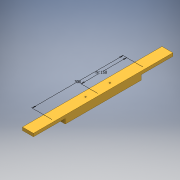
# Autodesk Inventor part: piXYstageStiltAttach
Saved by Autodesk Inventor 2016 (Build 200138000, 138)
## iProperties
Created: 2016-03-15
Part Number: piXYstageStiltAttach
Material: Generic
Document SubType Name: Modeling
Designer: sims01
Density: 1 g/cm^3
Appearance: Default
Author: sims01
Autodesk Inventor part; units mm, degrees
ref_plane "YZ Plane" through (0, 0, 0) normal (1, 0, 0) x (0, 1, 0)
ref_plane "XZ Plane" through (0, 0, 0) normal (0, 1, 0) x (-1, 0, 0)
ref_plane "XY Plane" through (0, 0, 0) normal (0, 0, 1) x (1, 0, 0)
sketch "Sketch1" plane through (0, 0, 0) normal (0, 0, 1) x (1, 0, 0)
  line L0 (-8, 55.5375) -> (8, 55.5375)
  line L1 (8, 55.5375) -> (8, -55.5375)
  line L2 (8, -55.5375) -> (-8, -55.5375)
  line L3 (-8, -55.5375) -> (-8, 55.5375)
  line L4 (-18, 229.9628) -> (18, 229.9628)
  line L5 (18, 229.9628) -> (18, -229.9628)
  line L6 (18, -229.9628) -> (-18, -229.9628)
  line L7 (-18, -229.9628) -> (-18, 229.9628)
  point P0 (0, 0)
  dimension "d0" = 16
  dimension "d1" = 111.075
  dimension "d2" = 55.5375
  dimension "d3" = 8
  dimension "d6" = 10
  dimension "d7" = 174.4253
  dimension "d8" = 10
  dimension "d9" = 174.4253
  constraints: 16 end point, 4 parallel, 2 horizontal, 2 perpendicular
  measures "d0" distance of L0.start L0.end
  measures "d1" distance of L0.end L1.end
  measures "d2" distance from line of point (0, 0) L0
  measures "d3" distance from line of point (0, 0) L1
  measures "d6" distance between parallel lines of L7 L3
  measures "d7" distance between parallel lines of L0 L4
  measures "d8" distance between parallel lines of L5 L1
  measures "d9" distance between parallel lines of L6 L2
sketch "Sketch2" plane through (0, 0, 0) normal (0, 0, 1) x (1, 0, 0)
  point P0 (0, 0)
  point P1 (0, 40)
  point P2 (0, -40)
  dimension "d4" = 80
  dimension "d5" = 40
  constraints: 2 vertical alignment
  measures "d4" distance of point (0, -40) point (0, 40)
  measures "d5" distance of point (0, 0) point (0, 40)
sketch "Sketch3" plane through (0, 0, 0) normal (0, 0, 1) x (1, 0, 0)
  point P0 (0, 0)
  point P1 (0, -150)
  point P2 (0, 150)
  dimension "d10" = 300
  dimension "d11" = 150
  constraints: 2 vertical alignment
  measures "d10" distance of point (0, 150) point (0, -150)
  measures "d11" distance of point (0, 0) point (0, 150)
extrude "baseExtrusion" add sketch "Sketch1" along normal blind 10 contours L0 L1 L2 L3 | L4 L5 L6 L7
hole "xyStageAttach_m5" at (0, 40, 0) at (0, -40, 0) direction (0, 0, 1) diameter 4.134 depth 14.2 tip angle 118 thread size "M5x0.8" class "6H" standard "ISO Metric profile"
sketch "Sketch4" plane through (0, 0, 0) normal (0, 0, -1) x (-1, 0, 0)
  line L0 (-18, 125) -> (18, 125)
  line L1 (18, 125) -> (18, -125)
  line L2 (18, -125) -> (-18, -125)
  line L3 (-18, -125) -> (-18, 125)
  line L4 (-18, 229.9628) -> (-18, -229.9628) projected
  line L5 (18, -229.9628) -> (18, 229.9628) projected
  point P0 (0, 0)
  dimension "d28" = 125
  dimension "d29" = 125
  constraints: 8 end point, 2 collinear, 2 parallel, 1 horizontal, 1 perpendicular
  measures "d28" distance from line of point (0, 0) L0
  measures "d29" distance from line of L2 point (0, 0)
extrude "Extrusion2" add sketch "Sketch4" along normal blind 16
sketch "Sketch5" plane through (0, 0, -16) normal (0, 0, -1) x (-1, 0, 0)
  line L0 (-10, -75) -> (10, -75)
  line L1 (10, -75) -> (10, 75)
  line L2 (10, 75) -> (-10, 75)
  line L3 (-10, 75) -> (-10, -75)
  point P0 (0, 0)
  dimension "d32" = 150
  dimension "d33" = 75
  dimension "d34" = 20
  dimension "d35" = 10
  constraints: 8 end point, 2 parallel, 1 horizontal, 1 perpendicular
  measures "d32" distance of L2.end L0.start
  measures "d33" distance from line of point (0, 0) L2
  measures "d34" distance of L1.end L2.end
  measures "d35" distance from line of point (0, 0) L3
extrude "Extrusion3" cut sketch "Sketch5" against normal blind 16
equation "\"d2\" = 0.5 * d1"
equation "\"d3\" = 0.5 * d0"
equation "\"d8\" = d6"
equation "\"d9\" = d7"
equation "\"d5\" = 0.5 * d4"
equation "\"d11\" = 0.5 * d10"
equation "\"d29\" = d28"
equation "\"d33\" = 0.5 * d32"
equation "\"d35\" = 0.5 * d34"
body "Solid1"
